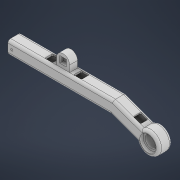
# Autodesk Inventor part: Fahrwerk_rocker_hinten
Saved by Autodesk Inventor 2021 (Build 250183000, 183)
## iProperties
Created: 2020-12-28
Part Number: Fahrwerk_rocker_hinten
Material: Generisch
Document SubType Name: Modeling
Designer: laure
Density: 1 g/cm^3
Appearance: Vorgabe
Author: laure
## iProperties of the stored document _3D-Druck.ipt
Created: 2021-01-24
Part Number: _3D-Druck
Material: Generisch
Document SubType Name: Modeling
Designer: laure
Density: 1 g/cm^3
Appearance: Vorgabe
Author: laure
Autodesk Inventor part; units mm, degrees
ref_plane "YZ Plane" through (0, 0, 0) normal (1, 0, 0) x (0, 1, 0)
ref_plane "XZ Plane" through (0, 0, 0) normal (0, 1, 0) x (-1, 0, 0)
ref_plane "XY Plane" through (0, 0, 0) normal (0, 0, 1) x (1, 0, 0)
sketch "Skizze1" plane through (0, 0, 0) normal (0, 0, 1) x (1, 0, 0)
  line L0 (-110, 10) -> (50, 10)
  line L1 (46.4735, -10) -> (-110, -10)
  line L2 (-153.2763, 0) -> (149.6579, 0) projected
  line L3 (99.5412, -29.3151) -> (46.4735, -10)
  line L4 (50, 10) -> (106.3816, -10.5212)
  line L5 (106.3816, -10.5212) -> (99.5412, -29.3151)
  line L6 (0, -37.1781) -> (0, 17.863) projected
  line L7 (-110, 10) -> (-110, -10)
  point P0 (0, 0)
  dimension "d5" = 20
  dimension "d56" = 0
  dimension "d57" = 0
  dimension "d58" = 60
  dimension "d138" = 160
  dimension "d140" = 20
  dimension "d141" = 10
  dimension "d142" = 110
  dimension "d143" = 50
  dimension "d144" = 10
  constraints: 12 end point, 2 parallel, 2 perpendicular, 1 horizontal, 1 other
  measures "d5" distance between parallel lines of L4 L3
  measures "d56" distance from line of L0 L4.start
  measures "d57" distance of L0.end L4.start
  measures "d58" distance from line of L4.start L5
  measures "d138" distance from line of L7 L0.end
  measures "d140" angle of L6 L5
  measures "d141" distance between parallel lines of L2 L0
  measures "d142" distance between parallel lines of L6 L7
  measures "d143" distance from line of point (50, 10) L6
  measures "d144" distance from line of point (50, 10) L2
sketch "Skizze4" plane through (0, 0, 0) normal (0, 0, 1) x (1, 0, 0)
  line L0 (-40, 10) -> (-20, 10)
  line L1 (-20, 10) -> (-20, 20)
  line L2 (-30, 30) -> (-30, 30)
  line L3 (-40, 20) -> (-40, 10)
  arc A0 (-30, 30) -> (-40, 20) centre (-30, 20) ccw
  arc A1 (-20, 20) -> (-30, 30) centre (-30, 20) ccw
  line L4 (-50.4853, 0) -> (8.4142, 0) projected
  line L5 (0, -6.4142) -> (0, 38.4853) projected
  line L6 (-35, 25) -> (-25, 25)
  line L7 (-25, 25) -> (-25, 15)
  line L8 (-25, 15) -> (-35, 15)
  line L9 (-35, 15) -> (-35, 25)
  line L10 (-35, 25) -> (-25, 15) construction
  line L11 (-25, 25) -> (-35, 15) construction
  point P0 (0, 0)
  point P1 (-30, 30)
  dimension "d74" = 20
  dimension "d75" = 20
  dimension "d78" = 10
  dimension "d116" = 10
  dimension "d160" = 10
  dimension "d161" = 10
  dimension "d162" = 20
  dimension "d167" = 10
  constraints: 20 end point, 4 parallel, 4 point on circle, 4 tangent, 2 centre point, 2 horizontal, 2 midpoint, 2 perpendicular, 1 concentric
  measures "d74" distance between parallel lines of L1 L3
  measures "d75" distance between parallel lines of L0 L2
  measures "d78" radius of A0
  measures "d116" distance between parallel lines of L0 L4
  measures "d160" distance of L7.end L8.end
  measures "d161" distance of L6.end L7.end
  measures "d162" distance between parallel lines of L5 L1
  measures "d167" distance from line of L0 A1.centre
extrude "Extrusion1" add sketch "Skizze1" against normal mid plane 20
sketch "Skizze13" plane through (0, 0, -10) normal (0, 0, -1) x (-1, 0, 0)
  line L0 (-106.3816, -10.5212) -> (-99.5412, -29.3151) projected
  circle A0 centre (-102.9614, -19.9181) radius 12.15
  circle A1 centre (-102.9614, -19.9181) radius 17
  point P0 (0, 0)
  point P1 (-105.5778, -12.7295)
  point P2 (-100.3449, -27.1068)
  dimension "d148" = 24.3
  dimension "d149" = 34
  constraints: 2 centre point, 1 coincident, 1 midpoint
  measures "d148" diameter of A0
  measures "d149" diameter of A1
extrude "Extrusion13" add sketch "Skizze13" against normal blind 20
extrude "Extrusion14" cut sketch "Skizze13" against normal up to surface (20 mm away) contours A0
shell "Wandung2" thickness 2.6 removed faces 1 at (-110, -3.3333, -3.3333)
extrude "Extrusion11" add sketch "Skizze4" against normal mid plane 12 contours L3 A0 A1 L1 L0 | L6 L7 L8 L9
sketch "Skizze12" plane through (0, 0, 10) normal (0, 0, 1) x (1, 0, 0)
  circle A0 centre (-104, 0) radius 1.6
  line L0 (-110, 6) -> (49.2947, 6) projected
  line L1 (-110, 10) -> (-110, -10) projected
  line L2 (50, 10) -> (-110, 10) projected
  point P0 (0, 0)
  point P1 (-110, -6)
  dimension "d133" = 3.2
  dimension "d135" = 6
  dimension "d147" = 10
  constraints: 1 centre point
  measures "d133" diameter of A0
  measures "d135" distance from line of L1 A0.centre
  measures "d147" distance from line of A0.centre L2
extrude "Extrusion12" cut sketch "Skizze12" against normal up to surface (20 mm away)
sketch "Skizze14" plane through (0, 0, 0) normal (0, 0, 1) x (1, 0, 0)
  circle A0 centre (102.9614, -19.9181) radius 12.15 projected
  circle A1 centre (102.9614, -19.9181) radius 9
  point P0 (0, 0)
  dimension "d157" = 18
  constraints: 1 centre point, 1 coincident
  measures "d157" diameter of A1
extrude "Extrusion15" add sketch "Skizze14" along normal mid plane 10
fillet "Rundung7" radius 4 10 edges at (71.7315, 2.0904, -10) (71.7315, 2.0904, 10) (-30, 10, 10) (-30, 10, -10) (-31.7633, -10, -10) (66.548, -17.3065, -10) (-31.7633, -10, 10) (66.548, -17.3065, 10) (118.9361, -25.7325, 10) (118.9361, -25.7325, -10)
sketch "Skizze17" plane through (-20, 10, 6) normal (0, 1, 0) x (1, 0, 0)
  line L0 (70, 0) -> (0, 0) projected
  line L1 (6, 0) -> (18, 0)
  line L2 (18, 0) -> (18, 12)
  line L3 (18, 12) -> (6, 12)
  line L4 (6, 12) -> (6, 0)
  line L5 (0, 0) -> (0, 12) projected
  line L6 (-90, 0) -> (66.4735, 0) projected
  line L7 (-38, 0) -> (-26, 0)
  line L8 (-26, 0) -> (-26, 12)
  line L9 (-26, 12) -> (-38, 12)
  line L10 (-38, 12) -> (-38, 0)
  line L11 (-20, 12) -> (-20, 0) projected
  point P0 (20, 6)
  point P1 (18, 0)
  point P2 (-26, 0)
  dimension "d176" = 12
  dimension "d177" = 12
  dimension "d178" = 6
  dimension "d179" = 12
  dimension "d180" = 12
  dimension "d181" = 6
  constraints: 16 end point, 4 parallel, 2 horizontal, 2 perpendicular, 2 point on line
  measures "d176" distance of L3.end L2.end
  measures "d177" distance of L2.end L1.end
  measures "d178" distance between parallel lines of L4 L5
  measures "d179" distance of L9.end L8.end
  measures "d180" distance of L8.end L7.end
  measures "d181" distance between parallel lines of L11 L8
extrude "Extrusion19" cut sketch "Skizze17" against normal blind 3
sketch "Skizze18" plane through (93.4629, -5.8192, 6) normal (0.3420201, 0.9396926, 0) x (0.9396926, -0.3420201, 0)
  line L0 (-42.7257, 0) -> (0, 0) projected
  line L1 (-18, 0) -> (-6, 0)
  line L2 (-6, 0) -> (-6, 12)
  line L3 (-6, 12) -> (-18, 12)
  line L4 (-18, 12) -> (-18, 0)
  line L5 (0, 0) -> (0, 12) projected
  point P0 (-89.8167, 6)
  point P1 (-6, 0)
  dimension "d184" = 12
  dimension "d185" = 12
  dimension "d186" = 6
  constraints: 8 end point, 2 parallel, 1 horizontal, 1 perpendicular, 1 point on line
  measures "d184" distance of L3.end L2.end
  measures "d185" distance of L2.end L1.end
  measures "d186" distance between parallel lines of L2 L5
extrude "Extrusion20" cut sketch "Skizze18" against normal blind 3
fillet "Rundung8" radius 2 12 edges at (-46, 8.7, -6) (-58, 8.7, -6) (-58, 8.7, 6) (-46, 8.7, 6) (-2, 8.7, 6) (-14, 8.7, -6) (-2, 8.7, -6) (-14, 8.7, 6) (76.1038, -0.8844, 6) (87.3801, -4.9887, 6) (87.3801, -4.9887, -6) (76.1038, -0.8844, -6)
extrude "Extrusion21" cut sketch "Skizze4" along normal up to surface (6 mm away) contours L6 L7 L8 L9
sketch "Skizze19" plane through (0, 0, -6) normal (0, 0, -1) x (-1, 0, 0)
  circle A0 centre (30, 20) radius 3.5
  line L0 (40, 10) -> (20, 10) projected
  line L1 (20, 20) -> (20, 10) projected
  point P0 (0, 0)
  dimension "d192" = 7
  dimension "d193" = 10
  dimension "d194" = 10
  constraints: 1 centre point
  measures "d192" diameter of A0
  measures "d193" distance from line of L0 A0.centre
  measures "d194" distance from line of L1 A0.centre
extrude "Extrusion22" cut sketch "Skizze19" against normal blind 3
sketch "Skizze20" plane through (-30, 20, -3) normal (0, 0, -1) x (-1, 0, 0)
  circle A0 centre (0, 0) radius 3.5 projected
  circle A1 centre (0, 0) radius 1.6
  point P0 (-30, -20)
  dimension "d197" = 3.2
  constraints: 1 centre point, 1 coincident
  measures "d197" diameter of A1
extrude "Extrusion23" cut sketch "Skizze20" against normal up to surface (3 mm away) contours A1
